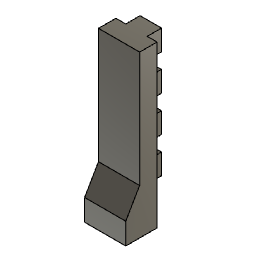
driver-cooler (Autodesk Fusion 360 design; units mm, degrees)
Autodesk Fusion 360 part; units mm, degrees
sketch "Sketch1" plane through (0, 0, 0) normal (0, 0, 1) x (1, 0, 0)
  line L0 (-10.5, 7.5) -> (10.5, 7.5)
  line L1 (10.5, 7.5) -> (10.5, -8)
  line L2 (10.5, -8) -> (-10.5, -8)
  line L3 (-10.5, -8) -> (-10.5, 7.5)
  line L4 (-11.5, -9) -> (-11.5, 8.5)
  line L5 (-11.5, 8.5) -> (11.5, 8.5)
  line L6 (11.5, 8.5) -> (11.5, -9)
  line L7 (11.5, -9) -> (-11.5, -9)
  dimension "d1" = 21
  dimension "d2" = 10.5
  dimension "d3" = 15.5
  dimension "d4" = 7.5
  dimension "d5" = -1
  constraint horizontal L0
  constraint vertical L1
  constraint horizontal L2
  constraint vertical L3
  measures "d1" distance of L1 L3
  measures "d2" distance of origin L1
  measures "d3" distance of L0 L2
  measures "d4" distance of origin L0
extrude "Extrude1" add sketch "Sketch1" along normal blind 95
sketch "Sketch2" plane through (0, 8.5, 0) normal (0, 1, 0) x (-1, 0, 0)
  line L0 (-11.5, 0) -> (11.5, 0)
  line L1 (11.5, 0) -> (11.5, 95)
  line L2 (11.5, 95) -> (-11.5, 95)
  line L3 (-11.5, 95) -> (-11.5, 0)
  line L4 (-5, 29) -> (5, 29)
  line L5 (5, 29) -> (5, 19.5)
  line L6 (5, 19.5) -> (-5, 19.5)
  line L7 (-5, 19.5) -> (-5, 29)
  line L8 (0, 0) -> (0, 45) construction
  line L9 (5, 39.5) -> (-5, 39.5)
  line L10 (-5, 39.5) -> (-5, 49)
  line L11 (-5, 49) -> (5, 49)
  line L12 (5, 49) -> (5, 39.5)
  line L13 (5, 59.5) -> (-5, 59.5)
  line L14 (-5, 59.5) -> (-5, 69)
  line L15 (-5, 69) -> (5, 69)
  line L16 (5, 69) -> (5, 59.5)
  line L17 (5, 79.5) -> (-5, 79.5)
  line L18 (-5, 79.5) -> (-5, 89)
  line L19 (-5, 89) -> (5, 89)
  line L20 (5, 89) -> (5, 79.5)
  dimension "d8" = 19.5
  dimension "d9" = 9.5
  dimension "d10" = 10
  dimension "d11" = 5
  dimension "d14" = 0
  dimension "d15" = 20
  constraint horizontal L4
  constraint vertical L5
  constraint horizontal L6
  constraint vertical L7
  constraint coincident L8.start origin
  constraint perpendicular L0 L8
  measures "d8" distance of L8.start L6
  measures "d9" distance of L4 L6
  measures "d10" distance of L5 L7
  measures "d11" distance of L7 L8
extrude "Extrude2" cut sketch "Sketch2" against normal up to surface (1 mm away) contours L4 L5 L6 L7 | L9 L10 L11 L12 | L13 L14 L15 L16 | L17 L18 L19 L20
sketch "Sketch3" plane through (0, 8.5, 0) normal (0, 1, 0) x (-1, 0, 0)
  line L0 (5, 69) -> (5, 59.5)
  line L1 (5, 59.5) -> (-5, 59.5)
  line L2 (-5, 59.5) -> (-5, 69)
  line L3 (-5, 69) -> (5, 69)
  line L4 (5, 49) -> (5, 39.5)
  line L5 (5, 39.5) -> (-5, 39.5)
  line L6 (-5, 39.5) -> (-5, 49)
  line L7 (-5, 49) -> (5, 49)
  line L8 (5, 89) -> (5, 79.5)
  line L9 (5, 79.5) -> (-5, 79.5)
  line L10 (-5, 79.5) -> (-5, 89)
  line L11 (-5, 89) -> (5, 89)
  line L12 (-5, 19.5) -> (-5, 29)
  line L13 (-5, 29) -> (5, 29)
  line L14 (5, 29) -> (5, 19.5)
  line L15 (5, 19.5) -> (-5, 19.5)
  line L16 (-11.5, 0) -> (11.5, 0)
  line L17 (11.5, 0) -> (11.5, 95)
  line L18 (11.5, 95) -> (-11.5, 95)
  line L19 (-11.5, 95) -> (-11.5, 0)
  line L20 (-5, 19.5) -> (5, 19.5)
  line L21 (5, 19.5) -> (5, 29)
  line L22 (5, 29) -> (-5, 29)
  line L23 (-5, 29) -> (-5, 19.5)
  line L24 (-6, 18.5) -> (6, 18.5)
  line L25 (6, 18.5) -> (6, 30)
  line L26 (6, 30) -> (-6, 30)
  line L27 (-6, 30) -> (-6, 18.5)
  line L28 (6, 38.5) -> (6, 50)
  line L29 (5, 49) -> (-5, 49)
  line L30 (-6, 38.5) -> (6, 38.5)
  line L31 (5, 39.5) -> (5, 49)
  line L32 (-5, 39.5) -> (5, 39.5)
  line L33 (-5, 49) -> (5, 49)
  line L34 (-5, 39.5) -> (-5, 49)
  line L35 (-5, 49) -> (-5, 39.5)
  line L36 (-6, 50) -> (-6, 38.5)
  line L37 (6, 50) -> (-6, 50)
  line L38 (5, 49) -> (5, 39.5)
  line L39 (5, 39.5) -> (-5, 39.5)
  line L40 (6, 58.5) -> (6, 70)
  line L41 (5, 69) -> (-5, 69)
  line L42 (-6, 58.5) -> (6, 58.5)
  line L43 (5, 59.5) -> (5, 69)
  line L44 (-5, 59.5) -> (5, 59.5)
  line L45 (-5, 69) -> (5, 69)
  line L46 (-5, 59.5) -> (-5, 69)
  line L47 (-5, 69) -> (-5, 59.5)
  line L48 (-6, 70) -> (-6, 58.5)
  line L49 (6, 70) -> (-6, 70)
  line L50 (5, 69) -> (5, 59.5)
  line L51 (5, 59.5) -> (-5, 59.5)
  line L52 (6, 78.5) -> (6, 90)
  line L53 (5, 89) -> (-5, 89)
  line L54 (-6, 78.5) -> (6, 78.5)
  line L55 (5, 79.5) -> (5, 89)
  line L56 (-5, 79.5) -> (5, 79.5)
  line L57 (-5, 89) -> (5, 89)
  line L58 (-5, 79.5) -> (-5, 89)
  line L59 (-5, 89) -> (-5, 79.5)
  line L60 (-6, 90) -> (-6, 78.5)
  line L61 (6, 90) -> (-6, 90)
  line L62 (5, 89) -> (5, 79.5)
  line L63 (5, 79.5) -> (-5, 79.5)
  dimension "d18" = 1
  dimension "d21" = 0
  dimension "d22" = 20
  constraint horizontal L20
  constraint vertical L21
  constraint horizontal L22
  constraint vertical L23
  constraint coincident L13.end L14.start
  constraint coincident L12.start L15.end
extrude "Extrude3" add sketch "Sketch3" along normal blind 8 contours L24 L25 L26 L27 | L28 L30 L36 L37 | L40 L42 L48 L49 | L52 L54 L60 L61
sketch "Sketch4" plane through (-11.5, 0, 0) normal (-1, 0, 0) x (0, -1, 0)
  line L0 (-8.5, 0) -> (9, 0)
  line L1 (9, 0) -> (9, 95)
  line L2 (9, 95) -> (-8.5, 95)
  line L3 (-8.5, 95) -> (-8.5, 0)
  line L4 (9, 95) -> (0.25, 95)
  line L5 (0.25, 95) -> (0.25, 25.1554)
  line L6 (9, 10) -> (9, 95)
  line L7 (9, 10) -> (0.25, 25.1554)
  dimension "d25" = 8.75
  dimension "d29" = 30
  dimension "d30" = 85
  constraint horizontal L4
  constraint vertical L5
  constraint vertical L6
  constraint coincident L1.end L2.start
  measures "d25" distance of L5 L6
  measures "d29" angle of L6 L7
  measures "d30" distance of L6.start L4
extrude "Extrude4" add sketch "Sketch4" against normal through all contours L1 L2 L4 L5 L6 L7
sketch "Sketch5" plane through (-11.5, 0, 0) normal (-1, 0, 0) x (0, -1, 0)
  line L0 (9, 95) -> (-8.5, 95)
  line L1 (-8.5, 95) -> (-8.5, 0)
  line L2 (-8.5, 0) -> (9, 0)
  line L3 (9, 0) -> (9, 95)
  line L4 (0.25, 95) -> (9, 95)
  line L5 (9, 10) -> (0.25, 25.1554)
  line L6 (0.25, 25.1554) -> (0.25, 95)
  line L7 (9, 95) -> (9, 10)
  line L8 (9.866, 10.5) -> (1.25, 25.4234)
  line L9 (1.25, 25.4234) -> (1.25, 95)
  dimension "d31" = 85
  dimension "d32" = 30
  dimension "d33" = 1
  constraint midpoint L0 L4.start
  constraint coincident L0.start L3.end
  constraint coincident L3 L5.start
  constraint perpendicular L0 L6
  measures "d31" distance of L4 L5.start
  measures "d32" angle of L5 L7
extrude "Extrude5" cut sketch "Sketch5" against normal through all contours L0 L3 L4 L7 L8 L9
sketch "Sketch6" plane through (-11.5, 0, 0) normal (-1, 0, 0) x (0, -1, 0)
  line L0 (9, 12) -> (1.25, 25.4234)
  line L1 (1.25, 25.4234) -> (1.25, 95)
  line L2 (1.25, 95) -> (-8.5, 95)
  line L3 (-8.5, 95) -> (-8.5, 0)
  line L4 (-8.5, 0) -> (9, 0)
  line L5 (9, 0) -> (9, 12)
  line L6 (-8.5, 95) -> (1.25, 95)
  line L7 (1.25, 95) -> (1.25, 90)
  line L8 (1.25, 90) -> (-8.5, 90)
  line L9 (-8.5, 90) -> (-8.5, 95)
  dimension "d35" = 5
  constraint horizontal L6
  constraint vertical L7
  constraint horizontal L8
  constraint vertical L9
  constraint coincident L1 L7.end
  constraint coincident L2.end L3.start
  measures "d35" distance of L6 L8
extrude "Extrude6" cut sketch "Sketch6" against normal through all contours L1 L2 L3 L6 L7 L8 L9
sketch "Sketch7" plane through (0, 0, 90) normal (0, 0, 1) x (-1, 0, 0)
  line L0 (-10.5, 0.25) -> (10.5, 0.25)
  line L1 (10.5, 0.25) -> (10.5, -7.5)
  line L2 (10.5, -7.5) -> (-10.5, -7.5)
  line L3 (-10.5, -7.5) -> (-10.5, 0.25)
  line L4 (-6, -8.5) -> (-6, -16.5)
  line L5 (-6, -16.5) -> (6, -16.5)
  line L6 (6, -16.5) -> (6, -8.5)
  line L7 (6, -8.5) -> (11.5, -8.5)
  line L8 (11.5, -8.5) -> (11.5, 1.25)
  line L9 (11.5, 1.25) -> (-11.5, 1.25)
  line L10 (-11.5, 1.25) -> (-11.5, -8.5)
  line L11 (-11.5, -8.5) -> (-6, -8.5)
extrude "Extrude7" add sketch "Sketch7" against normal blind 1 contours L0 L1 L2 L3
equation "d2 = ( 21 / 2 ) * 1 mm"
equation "d4 = ( 15 / 2 ) * 1 mm"
equation "d8 = 17 mm + 2.5 mm"
